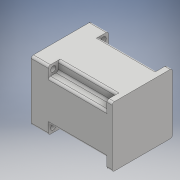
# Autodesk Inventor part: MOTOR
Saved by Autodesk Inventor 2018 (Build 220112000, 112)
## iProperties
Created: 2018-03-13
Part Number: MOTOR
Material: Generic
Document SubType Name: Modeling
Designer: m234547
Density: 1 g/cm^3
Appearance: Default
Author: m234547
Autodesk Inventor part; units mm, degrees
ref_plane "YZ Plane" through (0, 0, 0) normal (1, 0, 0) x (0, 1, 0)
ref_plane "XZ Plane" through (0, 0, 0) normal (0, 1, 0) x (-1, 0, 0)
ref_plane "XY Plane" through (0, 0, 0) normal (0, 0, 1) x (1, 0, 0)
sketch "Sketch1" plane through (0, 0, 0) normal (1, 0, 0) x (0, 1, 0)
  line L0 (28.3233, 27.0734) -> (-24.0767, 27.0734)
  line L1 (-26.0767, 25.0734) -> (-26.0767, -27.3266)
  line L2 (-24.0767, -29.3266) -> (28.3233, -29.3266)
  line L3 (30.3233, -27.3266) -> (30.3233, 25.0734)
  arc A0 (-24.0767, 27.0734) -> (-26.0767, 25.0734) centre (-24.0767, 25.0734) ccw
  arc A1 (30.3233, 25.0734) -> (28.3233, 27.0734) centre (28.3233, 25.0734) ccw
  arc A2 (28.3233, -29.3266) -> (30.3233, -27.3266) centre (28.3233, -27.3266) ccw
  arc A3 (-26.0767, -27.3266) -> (-24.0767, -29.3266) centre (-24.0767, -27.3266) ccw
  point P0 (0, 0)
  point P1 (30.3233, 27.0734)
  point P2 (-26.0767, -29.3266)
  point P3 (-26.0767, 27.0734)
  point P4 (30.3233, -29.3266)
  dimension "d0" = 56.4
  dimension "d1" = 56.4
  dimension "d18" = 2
  constraints: 8 end point, 8 point on circle, 8 point on line, 8 tangent, 4 centre point, 3 equal radius, 2 parallel, 1 horizontal, 1 perpendicular
  measures "d0" distance of point (30.323, -29.327) point (-26.077, -29.327)
  measures "d1" distance of point (-26.077, -29.327) point (-26.077, 27.073)
  measures "d18" radius of A0
extrude "Extrusion1" add sketch "Sketch1" along normal blind 16
sketch "Sketch5" plane through (16, 0, 0) normal (1, 0, 0) x (0, 0, -1)
  circle A0 centre (24.6966, 25.6933) radius 2.5
  circle A1 centre (24.6966, -21.4467) radius 2.5
  circle A2 centre (-22.4434, -21.4467) radius 2.5
  circle A3 centre (-22.4434, 25.6933) radius 2.5
  point P0 (0, 0)
  dimension "d38" = 5
  dimension "d39" = 5
  dimension "d40" = 5
  dimension "d41" = 5
  constraints: 4 centre point
  measures "d38" diameter of A0
  measures "d39" diameter of A1
  measures "d40" diameter of A2
  measures "d41" diameter of A3
extrude "Extrusion3" cut sketch "Sketch5" against normal blind 16
sketch "Sketch6" plane through (16, 0, 0) normal (1, 0, 0) x (0, 0, -1)
  line L0 (-25.0734, -26.0767) -> (27.3266, -26.0767) projected
  arc A0 (27.3266, -26.0767) -> (29.3266, -24.0767) centre (27.3266, -24.0767) ccw projected
  circle A1 centre (-22.4434, -21.4467) radius 2.5 projected
  circle A2 centre (24.6966, 25.6933) radius 2.5 projected
  circle A3 centre (24.6966, -21.4467) radius 2.5 projected
  circle A4 centre (-22.4434, 25.6933) radius 2.5 projected
  line L1 (-27.0734, 28.3233) -> (-27.0734, -24.0767) projected
  arc A5 (-27.0734, -24.0767) -> (-25.0734, -26.0767) centre (-25.0734, -24.0767) ccw projected
  line L2 (-25.0734, -26.0767) -> (27.3266, -26.0767) projected
  arc A6 (27.3266, -26.0767) -> (29.3266, -24.0767) centre (27.3266, -24.0767) ccw projected
  line L3 (29.3266, -24.0767) -> (29.3266, 28.3233) projected
  arc A7 (29.3266, 28.3233) -> (27.3266, 30.3233) centre (27.3266, 28.3233) ccw projected
  line L4 (27.3266, 30.3233) -> (-25.0734, 30.3233) projected
  arc A8 (-25.0734, 30.3233) -> (-27.0734, 28.3233) centre (-25.0734, 28.3233) ccw projected
  line L5 (20.0666, 30.3233) -> (20.0666, 21.0633)
  line L6 (20.0666, 21.0633) -> (29.3266, 21.0633)
  line L7 (20.0666, -26.0767) -> (20.0666, -16.8167)
  line L8 (20.0666, -16.8167) -> (29.3266, -16.8167)
  line L9 (-17.8134, 30.3233) -> (-17.8134, 21.0633)
  line L10 (-17.8134, 21.0633) -> (-27.0734, 21.0633)
  line L11 (-17.8134, -26.0767) -> (-17.8134, -16.8167)
  line L12 (-17.8134, -16.8167) -> (-27.0734, -16.8167)
  line L13 (29.3266, 21.0633) -> (29.3266, -16.8167)
  line L14 (20.0666, 30.3233) -> (-17.8134, 30.3233)
  line L15 (-25.0734, 30.3233) -> (27.3266, 30.3233) projected
  line L16 (-27.0734, 21.0633) -> (-27.0734, -16.8167)
  line L17 (-27.0734, -24.0767) -> (-27.0734, 28.3233) projected
  line L18 (20.0666, -26.0767) -> (-17.8134, -26.0767)
  line L19 (27.3266, -26.0767) -> (-25.0734, -26.0767) projected
  point P0 (0, 0)
  dimension "d44" = 9.26
  dimension "d45" = 9.26
  dimension "d46" = 9.26
  dimension "d47" = 9.26
  dimension "d48" = 9.26
  dimension "d49" = 9.26
  dimension "d50" = 9.26
  dimension "d51" = 9.26
  constraints: 24 end point, 4 collinear
  measures "d44" distance of L6.end L5.end
  measures "d45" distance of L5.end L5.start
  measures "d46" distance of L7.end L8.end
  measures "d47" distance of L7.start L7.end
  measures "d48" distance of L9.end L10.end
  measures "d49" distance of L9.start L9.end
  measures "d50" distance of L12.end L11.end
  measures "d51" distance of L11.end L11.start
extrude "Extrusion4" add sketch "Sketch6" along normal blind 55 contours L11 L12 L1 L10 L9 L4 L5 L6 L3 L8 L7 L0
sketch "Sketch7" plane through (71, 0, 0) normal (1, 0, 0) x (0, 0, -1)
  line L0 (27.3266, -26.0767) -> (-25.0734, -26.0767)
  line L1 (-27.0734, -24.0767) -> (-27.0734, 28.3233)
  line L2 (-25.0734, 30.3233) -> (27.3266, 30.3233)
  line L3 (29.3266, 28.3233) -> (29.3266, -24.0767)
  arc A0 (27.3266, -26.0767) -> (29.3266, -24.0767) centre (27.3266, -24.0767) ccw
  arc A1 (-27.0734, -24.0767) -> (-25.0734, -26.0767) centre (-25.0734, -24.0767) ccw
  arc A2 (-25.0734, 30.3233) -> (-27.0734, 28.3233) centre (-25.0734, 28.3233) ccw
  arc A3 (29.3266, 28.3233) -> (27.3266, 30.3233) centre (27.3266, 28.3233) ccw
  point P0 (0, 0)
  point P1 (-27.0734, 30.3233)
  point P2 (-27.0734, -26.0767)
  point P3 (29.3266, 30.3233)
  dimension "d54" = 56.4
  dimension "d55" = 56.4
  dimension "d56" = 2
  constraints: 8 end point, 8 point on circle, 8 tangent, 6 point on line, 4 centre point, 3 equal radius, 2 parallel, 1 horizontal, 1 perpendicular
  measures "d54" distance of point (-27.073, 30.323) point (29.327, 30.323)
  measures "d55" distance of point (-27.073, -26.077) point (-27.073, 30.323)
  measures "d56" radius of A0
extrude "Extrusion5" add sketch "Sketch7" along normal blind 5
fillet "Fillet1" radius 2 12 edges at (43.5, -16.8167, -29.3266) (43.5, -16.8167, -20.0666) (43.5, -26.0767, -20.0666) (43.5, -16.8167, 27.0734) (43.5, -16.8167, 17.8134) (43.5, -26.0767, 17.8134) (43.5, 21.0633, 27.0734) (43.5, 21.0633, 17.8134) (43.5, 30.3233, 17.8134) (43.5, 30.3233, -20.0666) (43.5, 21.0633, -20.0666) (43.5, 21.0633, -29.3266)
sketch "Sketch8" plane through (0, 0, 0) normal (-1, 0, 0) x (0, 0, 1)
  line L0 (-29.3266, 28.3233) -> (-29.3266, -24.0767) projected
  line L1 (-27.3266, -26.0767) -> (25.0734, -26.0767) projected
  line L2 (27.0734, -24.0767) -> (27.0734, 28.3233) projected
  line L3 (25.0734, 30.3233) -> (-27.3266, 30.3233) projected
  arc A0 (-27.3266, 30.3233) -> (-29.3266, 28.3233) centre (-27.3266, 28.3233) ccw projected
  arc A1 (27.0734, 28.3233) -> (25.0734, 30.3233) centre (25.0734, 28.3233) ccw projected
  arc A2 (25.0734, -26.0767) -> (27.0734, -24.0767) centre (25.0734, -24.0767) ccw projected
  circle A3 centre (-1.1266, 2.1233) radius 0.0027
  circle A4 centre (-1.1266, 2.1233) radius 19.05
  point P0 (0, 0)
  dimension "d60" = 38.1
  constraints: 2 centre point, 1 coincident
  measures "d60" diameter of A4
extrude "Extrusion6" add sketch "Sketch8" along normal blind 1.6
sketch "Sketch9" plane through (-1.6, 2.1233, -1.1266) normal (-1, 0, 0) x (0, 0, 1)
  circle A0 centre (0, 0) radius 3.175
  point P0 (1.1266, -2.1233)
  dimension "d63" = 6.35
  constraints: 1 centre point
  measures "d63" diameter of A0
extrude "Extrusion7" add sketch "Sketch9" along normal blind 20.6
sketch "Sketch10" plane through (0, 0, 0) normal (-1, 0, 0) x (0, 0, 1)
  point P0 (0, 0)
body "Solid1"
